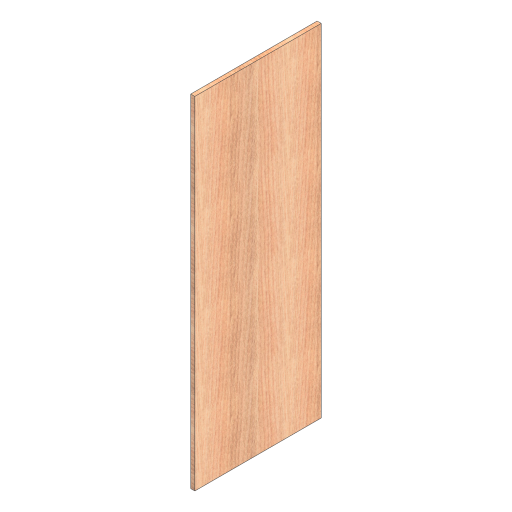
# Autodesk Inventor part: CUT PART R
Saved by Autodesk Inventor 2023.2 (Build 272271000, 271)
## iProperties
Created: 2022-12-01
Part Number: CUT PART R
Material: Wood (Birch)
Document SubType Name: Modeling
Designer: GUT
Mass: 2442 g
Surface Area: 7728.8 cm^2
Volume: 4440 cm^3
Density: 0.55 g/cm^3
Appearance: Birch - Natural Polished
Author: GUT
Autodesk Inventor part; units mm, degrees
ref_plane "YZ Plane" through (0, 0, 0) normal (1, 0, 0) x (0, 1, 0)
ref_plane "XZ Plane" through (0, 0, 0) normal (0, 1, 0) x (-1, 0, 0)
ref_plane "XY Plane" through (0, 0, 0) normal (0, 0, 1) x (1, 0, 0)
sketch "Sketch1" plane through (0, 0, 0) normal (1, 0, 0) x (0, 1, 0)
  line L0 (-666.0177, 341.6224) -> (333.9823, 341.6224)
  line L1 (333.9823, 341.6224) -> (333.9823, -28.3776)
  line L2 (333.9823, -28.3776) -> (-666.0177, -28.3776)
  line L3 (-666.0177, -28.3776) -> (-666.0177, 341.6224)
  point P0 (0, 0)
  dimension "d0" = 370
  dimension "d1" = 1000
  constraints: 8 end point, 2 parallel, 1 horizontal, 1 perpendicular
  measures "d0" distance of L0.end L1.end
  measures "d1" distance of L0.start L0.end
extrude "Extrusion1" add sketch "Sketch1" along normal blind 12
body "Solid1"
